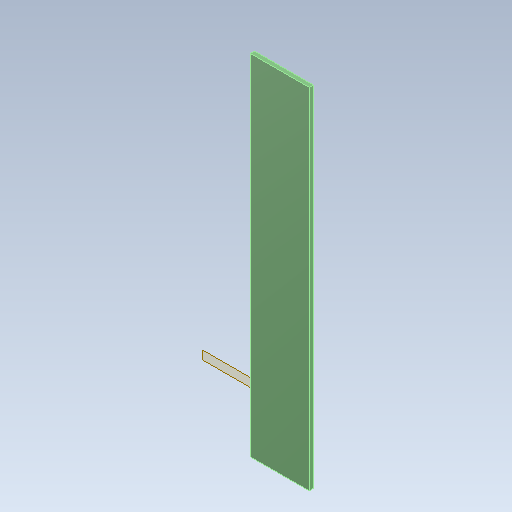
# Autodesk Inventor part: pcd stand in
Saved by Autodesk Inventor 2021 (Build 250183000, 183)
## iProperties
Created: 2020-09-26
Part Number: pcd stand in
Material: Generic
Document SubType Name: Modeling
Designer: capta
Density: 1 g/cm^3
Appearance: Smooth - Dark Forest Green
Author: capta
Autodesk Inventor part; units mm, degrees
ref_plane "YZ Plane" through (0, 0, 0) normal (1, 0, 0) x (0, 1, 0)
ref_plane "XZ Plane" through (0, 0, 0) normal (0, 1, 0) x (-1, 0, 0)
ref_plane "XY Plane" through (0, 0, 0) normal (0, 0, 1) x (1, 0, 0)
ref_plane "Work Plane1" through (0, 0, 0) normal (0, 0, 1) x (1, 0, 0)
sketch "Sketch1" plane through (0, 0, 0) normal (0, 0, 1) x (1, 0, 0)
  line L0 (41.8295, 113.9719) -> (18.9695, 113.9719)
  line L1 (18.9695, 113.9719) -> (18.9695, -21.8882)
  line L2 (18.9695, -21.8882) -> (41.8295, -21.8882)
  line L3 (41.8295, -21.8882) -> (41.8295, 113.9719)
  line L4 (41.8295, 113.9719) -> (18.9695, -21.8882) construction
  line L5 (18.9695, 113.9719) -> (41.8295, -21.8882) construction
  point P0 (0, 0)
  point P1 (30.3995, 46.0418)
  dimension "d0" = 22.86
  dimension "d1" = 135.86
  constraints: 12 end point, 2 midpoint, 2 parallel, 1 horizontal, 1 perpendicular
  measures "d0" distance of L1.end L2.end
  measures "d1" distance of L2.end L0.start
extrude "Extrusion1" add sketch "Sketch1" along normal blind 1.6256
body "Solid1"
